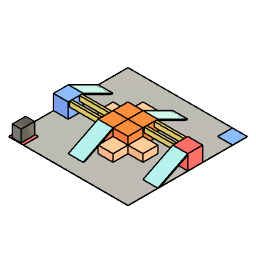
CRTC 2025 比赛场地 v4 (Autodesk Fusion 360 design; units mm, degrees)
Autodesk Fusion 360 part; units mm, degrees
sketch "草图1" plane through (0, 0, 0) normal (0, 0, 1) x (1, 0, 0)
  line L0 (0, 0) -> (2400, 0)
  line L1 (2400, 0) -> (2400, 2400)
  line L2 (2400, 2400) -> (0, 2400)
  line L3 (0, 2400) -> (0, 0)
  line L4 (0, 0) -> (300, 0)
  line L5 (0, 300) -> (0, 0)
  line L6 (300, 300) -> (300, 0)
  line L7 (300, 0) -> (600, 0)
  line L8 (600, 300) -> (600, 0)
  line L9 (600, 0) -> (900, 0)
  line L10 (900, 300) -> (900, 0)
  line L11 (900, 0) -> (1200, 0)
  line L12 (1200, 300) -> (1200, 0)
  line L13 (1200, 0) -> (1500, 0)
  line L14 (1500, 300) -> (1500, 0)
  line L15 (1500, 0) -> (1800, 0)
  line L16 (1800, 300) -> (1800, 0)
  line L17 (1800, 0) -> (2100, 0)
  line L18 (2100, 300) -> (2100, 0)
  line L19 (2100, 0) -> (2400, 0)
  line L20 (0, 600) -> (0, 300)
  line L21 (0, 300) -> (300, 300)
  line L22 (300, 600) -> (300, 300)
  line L23 (300, 300) -> (600, 300)
  line L24 (600, 600) -> (600, 300)
  line L25 (600, 300) -> (900, 300)
  line L26 (900, 600) -> (900, 300)
  line L27 (900, 300) -> (1200, 300)
  line L28 (1200, 600) -> (1200, 300)
  line L29 (1200, 300) -> (1500, 300)
  line L30 (1500, 600) -> (1500, 300)
  line L31 (1500, 300) -> (1800, 300)
  line L32 (1800, 600) -> (1800, 300)
  line L33 (1800, 300) -> (2100, 300)
  line L34 (2100, 600) -> (2100, 300)
  line L35 (2100, 300) -> (2400, 300)
  line L36 (0, 900) -> (0, 600)
  line L37 (0, 600) -> (300, 600)
  line L38 (300, 900) -> (300, 600)
  line L39 (300, 600) -> (600, 600)
  line L40 (600, 900) -> (600, 600)
  line L41 (600, 600) -> (900, 600)
  line L42 (900, 900) -> (900, 600)
  line L43 (900, 600) -> (1200, 600)
  line L44 (1200, 900) -> (1200, 600)
  line L45 (1200, 600) -> (1500, 600)
  line L46 (1500, 900) -> (1500, 600)
  line L47 (1500, 600) -> (1800, 600)
  line L48 (1800, 900) -> (1800, 600)
  line L49 (1800, 600) -> (2100, 600)
  line L50 (2100, 900) -> (2100, 600)
  line L51 (2100, 600) -> (2400, 600)
  line L52 (0, 1200) -> (0, 900)
  line L53 (0, 900) -> (300, 900)
  line L54 (300, 1200) -> (300, 900)
  line L55 (300, 900) -> (600, 900)
  line L56 (600, 1200) -> (600, 900)
  line L57 (600, 900) -> (900, 900)
  line L58 (900, 1200) -> (900, 900)
  line L59 (900, 900) -> (1200, 900)
  line L60 (1200, 1200) -> (1200, 900)
  line L61 (1200, 900) -> (1500, 900)
  line L62 (1500, 1200) -> (1500, 900)
  line L63 (1500, 900) -> (1800, 900)
  line L64 (1800, 1200) -> (1800, 900)
  line L65 (1800, 900) -> (2100, 900)
  line L66 (2100, 1200) -> (2100, 900)
  line L67 (2100, 900) -> (2400, 900)
  line L68 (0, 1500) -> (0, 1200)
  line L69 (0, 1200) -> (300, 1200)
  line L70 (300, 1500) -> (300, 1200)
  line L71 (300, 1200) -> (600, 1200)
  line L72 (600, 1500) -> (600, 1200)
  line L73 (600, 1200) -> (900, 1200)
  line L74 (900, 1500) -> (900, 1200)
  line L75 (900, 1200) -> (1200, 1200)
  line L76 (1200, 1500) -> (1200, 1200)
  line L77 (1200, 1200) -> (1500, 1200)
  line L78 (1500, 1500) -> (1500, 1200)
  line L79 (1500, 1200) -> (1800, 1200)
  line L80 (1800, 1500) -> (1800, 1200)
  line L81 (1800, 1200) -> (2100, 1200)
  line L82 (2100, 1500) -> (2100, 1200)
  line L83 (2100, 1200) -> (2400, 1200)
  line L84 (0, 1800) -> (0, 1500)
  line L85 (0, 1500) -> (300, 1500)
  line L86 (300, 1800) -> (300, 1500)
  line L87 (300, 1500) -> (600, 1500)
  line L88 (600, 1800) -> (600, 1500)
  line L89 (600, 1500) -> (900, 1500)
  line L90 (900, 1800) -> (900, 1500)
  line L91 (900, 1500) -> (1200, 1500)
  line L92 (1200, 1800) -> (1200, 1500)
  line L93 (1200, 1500) -> (1500, 1500)
  line L94 (1500, 1800) -> (1500, 1500)
  line L95 (1500, 1500) -> (1800, 1500)
  line L96 (1800, 1800) -> (1800, 1500)
  line L97 (1800, 1500) -> (2100, 1500)
  line L98 (2100, 1800) -> (2100, 1500)
  line L99 (2100, 1500) -> (2400, 1500)
  line L100 (0, 2100) -> (0, 1800)
  line L101 (0, 1800) -> (300, 1800)
  line L102 (300, 2100) -> (300, 1800)
  line L103 (300, 1800) -> (600, 1800)
  line L104 (600, 2100) -> (600, 1800)
  line L105 (600, 1800) -> (900, 1800)
  line L106 (900, 2100) -> (900, 1800)
  line L107 (900, 1800) -> (1200, 1800)
  line L108 (1200, 2100) -> (1200, 1800)
  line L109 (1200, 1800) -> (1500, 1800)
  line L110 (1500, 2100) -> (1500, 1800)
  line L111 (1500, 1800) -> (1800, 1800)
  line L112 (1800, 2100) -> (1800, 1800)
  line L113 (1800, 1800) -> (2100, 1800)
  line L114 (2100, 2100) -> (2100, 1800)
  line L115 (2100, 1800) -> (2400, 1800)
  line L116 (0, 2400) -> (0, 2100)
  line L117 (0, 2100) -> (300, 2100)
  line L118 (300, 2400) -> (300, 2100)
  line L119 (300, 2100) -> (600, 2100)
  line L120 (600, 2400) -> (600, 2100)
  line L121 (600, 2100) -> (900, 2100)
  line L122 (900, 2400) -> (900, 2100)
  line L123 (900, 2100) -> (1200, 2100)
  line L124 (1200, 2400) -> (1200, 2100)
  line L125 (1200, 2100) -> (1500, 2100)
  line L126 (1500, 2400) -> (1500, 2100)
  line L127 (1500, 2100) -> (1800, 2100)
  line L128 (1800, 2400) -> (1800, 2100)
  line L129 (1800, 2100) -> (2100, 2100)
  line L130 (2100, 2400) -> (2100, 2100)
  line L131 (2100, 2100) -> (2400, 2100)
  dimension "d1" = 2400
  dimension "d2" = 2400
  dimension "d3" = 300
  dimension "d4" = 300
  dimension "d7" = 2100
  dimension "d8" = 2100
  constraint horizontal L0
  constraint vertical L1
  constraint horizontal L2
  constraint vertical L3
  constraint coincident L0.start L3.end
  constraint horizontal L4
  constraint vertical L5
  measures "d1" distance of L0.start L0.end
  measures "d2" distance of L0.start L2.end
  measures "d3" distance of L0.start L4.end
  measures "d4" distance of L0.start L5.start
extrude "拉伸1" add sketch "草图1" against normal blind 6 makes body 1
extrude "拉伸2" add sketch "草图1" along normal blind 300 separate body contours L58 L59 L60 L75 makes body 2
extrude "拉伸3" add sketch "草图1" along normal blind 300 separate body contours L74 L75 L76 L91 makes body 3
extrude "拉伸4" add sketch "草图1" along normal blind 300 separate body contours L76 L77 L78 L93 makes body 4
extrude "拉伸5" add sketch "草图1" along normal blind 300 separate body contours L60 L61 L62 L77 makes body 5
extrude "拉伸6" add sketch "草图1" along normal blind 300 separate body contours L3 L52 L53 L54 L69 | L1 L82 L83 L99 makes body 6 at (0, 1100, 100) makes body 7 at (2100, 1400, 100)
extrude "拉伸7" add sketch "草图1" along normal blind 150 separate body contours L44 L45 L46 L61 | L72 L73 L74 L89 | L62 L63 L64 L79 | L90 L91 L92 L107 makes body 9 at (1300, 800, 0) makes body 9 at (1600, 1100, 0) makes body 8 at (700, 1400, 0) makes body 8 at (1000, 1700, 0)
extrude "拉伸8" add sketch "草图1" along normal blind 300 separate body contours L1 L50 L51 L67 | L1 L66 L67 L83 makes body 10
sketch "草图2" plane through (2400, 0, 0) normal (1, 0, 0) x (0, 1, 0)
  line L0 (600, 0) -> (1200, 0)
  line L1 (1200, 0) -> (1200, 300)
  line L2 (1200, 300) -> (600, 300)
  line L3 (600, 300) -> (600, 0)
  line L4 (600, 0) -> (1200, 300)
  line L5 (1200, 300) -> (1208.9443, 282.1115)
  line L6 (1208.9443, 282.1115) -> (644.7214, 0)
  dimension "d30" = 20
  constraint coincident L0.start L3.end
  constraint coincident L1.end L2.start
  constraint perpendicular L4 L5
  constraint coincident L0 L6.end
  constraint perpendicular L5 L6
  measures "d30" distance of L1.end L5.end
extrude "拉伸9" cut sketch "草图2" against normal blind 300 contours L2 L3 L4 | L0 L1 L6 bodies 10
copy_body "复制和粘贴实体1" bodies 10 makes body 11
move_body "移动1" bodies 11 to x (1, 0, 0) y (0, 1, 0) z (0, 0, 1) at (-1200, -300, 0)
pattern_circular "C-阵列1" count 2 over 360 about axis through (1200, 1200, 0) along (0, 0, 1) of bodies 10 11 makes body 12 at (100, 1600, 100) makes body 13 at (1300, 1900, 100)
ref_plane "工作平面1" through (750, 1050, 75) normal (0, -1, 0) x (1, 0, 0)
ref_plane "工作平面2" through (750, 950, 75) normal (0, -1, 0) x (1, 0, 0)
ref_plane "工作平面3" through (750, 925, 75) normal (0, -1, 0) x (1, 0, 0)
sketch "草图3" plane through (0, 925, 0) normal (0, -1, 0) x (-1, 0, 0)
  line L0 (-900, -300) -> (-300, -300)
  line L1 (-300, -300) -> (-300, -200)
  line L2 (-300, -200) -> (-900, -200)
  line L3 (-900, -200) -> (-900, -300)
  dimension "d34" = 100
  constraint horizontal L0
  constraint perpendicular L0 L1
  constraint perpendicular L1 L2
  constraint perpendicular L0 L3
  measures "d34" distance of L0.end L1.end
sketch "草图4" plane through (0, 925, 0) normal (0, -1, 0) x (-1, 0, 0)
extrude "拉伸10" add sketch "草图3" against normal blind 50 separate body makes body 14
mirror "镜像1" about plane through (750, 1050, 75) normal (0, -1, 0) of bodies 14 makes body 15
pattern_circular "C-阵列2" count 2 over 360 about axis through (1200, 1200, 0) along (0, 0, 1) of bodies 15 14 makes body 16 at (1700, 1475, 233.3333) makes body 17 at (1700, 1225, 233.3333)
sketch "草图5" plane through (0, 0, 0) normal (0, 0, 1) x (-1, 0, 0)
  line L0 (0, -2400) -> (0, 0)
  line L1 (0, 0) -> (-2400, 0)
  line L2 (-2400, 0) -> (-2400, -2400)
  line L3 (-2400, -2400) -> (0, -2400)
  line L4 (0, 0) -> (-300, 0)
  line L5 (-300, 0) -> (-300, -300)
  line L6 (-300, -300) -> (0, -300)
  line L7 (0, -300) -> (0, 0)
  line L8 (-2400, -2400) -> (-2100, -2400)
  line L9 (-2100, -2400) -> (-2100, -2100)
  line L10 (-2100, -2100) -> (-2400, -2100)
  line L11 (-2400, -2100) -> (-2400, -2400)
  dimension "d41" = 300
  dimension "d42" = 300
  dimension "d43" = 300
  dimension "d44" = 300
  constraint horizontal L4
  constraint vertical L5
  constraint horizontal L6
  constraint vertical L7
  constraint coincident L0.end L1.start
  constraint horizontal L8
  constraint vertical L9
  constraint horizontal L10
  constraint vertical L11
  constraint coincident L2.end L3.start
  measures "d41" distance of L0.end L4.end
  measures "d42" distance of L0.end L6.end
  measures "d43" distance of L2.end L8.end
  measures "d44" distance of L2.end L10.end
sketch "草图6" plane through (0, 0, 0) normal (0, 0, 1) x (-1, 0, 0)
  line L0 (0, -300) -> (-300, 0)
  line L1 (-300, -300) -> (0, 0)
  line L2 (-60, -15) -> (-240, -15)
  line L3 (-240, -15) -> (-240, -285)
  line L4 (-240, -285) -> (-60, -285)
  line L5 (-60, -285) -> (-60, -15)
  line L6 (-60, -15) -> (-240, -285) construction
  line L7 (-240, -15) -> (-60, -285) construction
  point P0 (-150, -150)
  dimension "d45" = 180
  dimension "d46" = 270
  constraint coincident L1.end origin
  constraint perpendicular L0 L1
  constraint horizontal L2
  constraint perpendicular L2 L3
  constraint parallel L2 L4
  constraint parallel L3 L5
  constraint coincident L6 P0
  constraint coincident L7 P0
  constraint midpoint L1 P0
  measures "d45" distance of L3.end L4.end
  measures "d46" distance of L2.end L3.end
extrude "拉伸11" add sketch "草图6" along normal blind 240 separate body makes body 18
extrude "拉伸12" cut sketch "草图5" against normal blind 1 contours L0 L1 L4 L5 L6 L7 | L2 L3 L8 L9 L10 L11 bodies 1
extrude "拉伸13" add sketch "草图5" against normal blind 1 separate body contours L0 L1 L4 L5 L6 L7 | L2 L3 L8 L9 L10 L11 makes body 19 at (100, 200, 0) makes body 20 at (2200, 2300, 0)
named bodies: "底层泡沫", "中央高台3", "中央高台2", "中央高台1", "中央高台4", "蓝方启动高台", "红方启动高台", "蓝方台阶", "红方台阶", "红方高台坡道", "红方中央高台坡道", "蓝方高台坡道", "蓝方中央高台坡道", "蓝方右桥梁", "蓝方左桥梁", "红方右桥梁", "红方左桥梁", "机器人最大尺寸", "红方启动区", "蓝方启动区"
